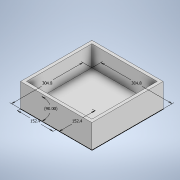
# Autodesk Inventor part: Box with dimensions
Saved by Autodesk Inventor 2020 (Build 240168000, 168)
## iProperties
Created: 2020-01-10
Part Number: Box with dimensions
Material: Generic
Document SubType Name: Modeling
Designer: ColinP
Density: 1 g/cm^3
Appearance: Default
Author: ColinP
Autodesk Inventor part; units mm, degrees
ref_plane "YZ Plane" through (0, 0, 0) normal (1, 0, 0) x (0, 1, 0)
ref_plane "XZ Plane" through (0, 0, 0) normal (0, 1, 0) x (-1, 0, 0)
ref_plane "XY Plane" through (0, 0, 0) normal (0, 0, 1) x (1, 0, 0)
sketch "Sketch1" plane through (0, 0, 0) normal (0, 1, 0) x (-1, 0, 0)
  line L0 (0, 0) -> (0, 152.4)
  line L1 (0, 152.4) -> (152.4, 152.4)
  line L2 (152.4, 152.4) -> (152.4, -152.4)
  line L3 (152.4, -152.4) -> (-152.4, -152.4)
  line L4 (-152.4, -152.4) -> (-152.4, 152.4)
  line L5 (-152.4, 152.4) -> (0, 152.4)
  dimension "d0" = 152.4
  dimension "d1" = 152.4
  dimension "d2" = 304.8
  dimension "d3" = 90
  dimension "d4" = 304.8
  constraints: 12 end point, 5 perpendicular, 1 point on line, 1 vertical
  measures "d0" distance of L0.start L0.end
  measures "d1" distance of L0.end L1.end
  measures "d2" distance of L1.end L2.end
  measures "d3" angle of L1 L2
  measures "d4" distance of L2.end L3.end
extrude "Extrusion1" add sketch "Sketch1" along normal blind 12.7
sketch "Sketch2" plane through (0, 12.7, 0) normal (0, 1, 0) x (1, 0, 0)
  line L0 (-152.4, -152.4) -> (152.4, -152.4) projected
  line L1 (-152.4, -152.4) -> (-152.4, -139.7)
  line L2 (-152.4, 152.4) -> (-152.4, -152.4) projected
  line L3 (-152.4, -139.7) -> (152.4, -139.7)
  line L4 (152.4, -152.4) -> (152.4, 152.4) projected
  line L5 (152.4, -139.7) -> (139.7, -139.7)
  line L6 (139.7, -139.7) -> (139.7, 139.7)
  line L7 (139.7, 139.7) -> (-139.7, 139.7)
  line L8 (-139.7, 139.7) -> (-139.7, -139.7)
  line L9 (152.4, 152.4) -> (-152.4, 152.4) projected
  point P0 (0, 0)
  dimension "d7" = 12.7
  dimension "d8" = 304.8
  dimension "d9" = 12.7
  dimension "d10" = 279.4
  dimension "d11" = 279.4
  dimension "d12" = 90
  dimension "d13" = 279.4
  constraints: 12 end point, 4 point on line, 2 perpendicular
  measures "d7" distance of L0.start L1.end
  measures "d8" distance of L1.end L3.end
  measures "d9" distance of L3.end L5.end
  measures "d10" distance of L5.end L6.end
  measures "d11" distance of L6.end L7.end
  measures "d12" angle of L7 L6
  measures "d13" distance of L7.end L8.end
extrude "Extrusion2" add sketch "Sketch2" along normal blind 88.9 contours L1 L3 L4 L0 | L2 L9 L4 L3 L6 L7 L8
body "Solid1"
